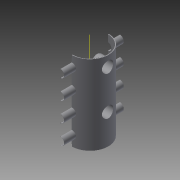
# Autodesk Inventor part: Detection Region Vacuum Collar v2
Saved by Autodesk Inventor 2015 (Build 190159000, 159)
## iProperties
Created: 2014-06-20
Part Number: Detection Region Vacuum Collar v2
Material: Generic
Document SubType Name: Modeling
Designer: Aki
Density: 1 g/cm^3
Appearance: Default
Author: Aki
Autodesk Inventor part; units mm, degrees
ref_plane "XZ Plane" through (0, 0, 0) normal (0, 1, 0) x (-1, 0, 0)
sketch "Sketch1" plane through (0, 0, 0) normal (0, 1, 0) x (-1, 0, 0)
  circle A0 centre (0, 0) radius 101.6
  circle A1 centre (0, 0) radius 97.6
  dimension "d0" = 203.2
  dimension "d3" = 195.2
  constraints: 2 centre point, 2 coincident
  measures "d0" diameter of A0
  measures "d3" diameter of A1
extrude "Extrusion2" add sketch "Sketch1" along normal blind 437.1
ref_plane "Work Plane1" through (0, 0, 101.6) normal (0, 0, 1) x (1, 0, 0)
sketch "Sketch2" plane through (0, 0, 101.6) normal (0, 0, 1) x (1, 0, 0)
  circle A0 centre (0, 57.3) radius 22.25
  circle A1 centre (0, 164.8) radius 22.25
  circle A2 centre (0, 272.3) radius 22.25
  circle A3 centre (0, 379.8) radius 22.25
  line L0 (101.6, 437.1) -> (-101.6, 437.1) projected
  line L1 (-101.6, 0) -> (101.6, 0) projected
  point P0 (0, 0)
  dimension "d7" = 44.5
  dimension "d8" = 44.5
  dimension "d9" = 44.5
  dimension "d10" = 44.5
  dimension "d11" = 57.3
  dimension "d12" = 57.3
  dimension "d13" = 215
  dimension "d14" = 215
  constraints: 4 centre point
  measures "d7" diameter of A0
  measures "d8" diameter of A1
  measures "d9" diameter of A2
  measures "d10" diameter of A3
  measures "d11" distance from line of L0 A3.centre
  measures "d12" distance from line of L1 A0.centre
  measures "d13" distance of A2.centre A0.centre
  measures "d14" distance of A3.centre A1.centre
extrude "Extrusion8" add sketch "Sketch2" against normal up to next
sketch "Sketch13" plane through (0, 0, 101.6) normal (0, 0, 1) x (1, 0, 0)
  circle A0 centre (0, 57.3) radius 22.25
  circle A1 centre (0, 164.8) radius 22.25
  circle A2 centre (0, 272.3) radius 22.25
  circle A3 centre (0, 379.8) radius 22.25
  line L0 (101.6, 437.1) -> (-101.6, 437.1) projected
  line L1 (-101.6, 0) -> (101.6, 0) projected
  point P0 (0, 0)
  dimension "d104" = 44.5
  dimension "d105" = 44.5
  dimension "d106" = 44.5
  dimension "d107" = 44.5
  dimension "d108" = 57.3
  dimension "d109" = 57.3
  dimension "d110" = 215
  dimension "d111" = 215
  constraints: 4 centre point
  measures "d104" diameter of A0
  measures "d105" diameter of A1
  measures "d106" diameter of A2
  measures "d107" diameter of A3
  measures "d108" distance from line of L0 A3.centre
  measures "d109" distance from line of L1 A0.centre
  measures "d110" distance of A2.centre A0.centre
  measures "d111" distance of A3.centre A1.centre
extrude "Extrusion9" add sketch "Sketch13" along normal blind 62.5
ref_plane "Work Plane2" through (0, 0, -101.6) normal (0, 0, 1) x (1, 0, 0)
sketch "Sketch3" plane through (0, 0, -101.6) normal (0, 0, 1) x (1, 0, 0)
  circle A0 centre (0, 57.3) radius 22.25
  circle A1 centre (0, 164.8) radius 22.25
  circle A2 centre (0, 272.3) radius 22.25
  circle A3 centre (0, 379.8) radius 22.25
  line L0 (101.6, 437.1) -> (-101.6, 437.1) projected
  line L1 (-101.6, 0) -> (101.6, 0) projected
  line L2 (0, 357.55) -> (0, 402.05) projected
  point P0 (0, 0)
  dimension "d18" = 44.5
  dimension "d19" = 44.5
  dimension "d20" = 44.5
  dimension "d21" = 44.5
  dimension "d22" = 57.3
  dimension "d23" = 57.3
  dimension "d24" = 215
  dimension "d25" = 215
  dimension "d26" = 0
  constraints: 4 centre point
  measures "d18" diameter of A0
  measures "d19" diameter of A1
  measures "d20" diameter of A2
  measures "d21" diameter of A3
  measures "d22" distance from line of L0 A3.centre
  measures "d23" distance from line of L1 A0.centre
  measures "d24" distance of A0.centre A2.centre
  measures "d25" distance of A3.centre A1.centre
  measures "d26" distance from line of L2 A3.centre
extrude "Extrusion10" add sketch "Sketch3" along normal up to next
sketch "Sketch14" plane through (0, 0, -101.6) normal (0, 0, 1) x (1, 0, 0)
  circle A0 centre (0, 57.3) radius 22.25
  circle A1 centre (0, 164.8) radius 22.25 projected
  circle A2 centre (0, 164.8) radius 22.25
  circle A3 centre (0, 272.3) radius 22.25
  circle A4 centre (0, 379.8) radius 22.25
  line L0 (-101.6, 0) -> (101.6, 0) projected
  line L1 (101.6, 437.1) -> (-101.6, 437.1) projected
  point P0 (0, 0)
  dimension "d116" = 44.5
  dimension "d117" = 44.5
  dimension "d118" = 44.5
  dimension "d119" = 44.5
  dimension "d120" = 57.3
  dimension "d121" = 215
  dimension "d122" = 215
  dimension "d123" = 57.3
  constraints: 4 centre point, 1 coincident
  measures "d116" diameter of A0
  measures "d117" diameter of A2
  measures "d118" diameter of A3
  measures "d119" diameter of A4
  measures "d120" distance from line of L0 A0.centre
  measures "d121" distance of A3.centre A0.centre
  measures "d122" distance of A4.centre A2.centre
  measures "d123" distance from line of L1 A4.centre
extrude "Extrusion11" add sketch "Sketch14" against normal blind 62.5
sketch "Sketch15" plane through (0, 379.8, -164.1) normal (0, 0, -1) x (-1, 0, 0)
  circle A0 centre (0, -322.5106) radius 21.35
  point P0 (0, -379.8)
  dimension "d126" = 42.7
  constraints: 1 centre point
  measures "d126" diameter of A0
hole "Hole8" at (0, 57.2894, -164.1) direction (0, 0, 1) diameter 42.7 end through all
sketch "Sketch16" plane through (0, 164.8, -164.1) normal (0, 0, -1) x (-1, 0, 0)
  circle A0 centre (0, 0) radius 21.35
  point P0 (0, -164.8)
  dimension "d134" = 42.7
  constraints: 1 centre point
  measures "d134" diameter of A0
hole "Hole9" at (0, 164.8, -164.1) direction (0, 0, 1) diameter 42.7 end through all
sketch "Sketch17" plane through (0, 272.3, -164.1) normal (0, 0, -1) x (-1, 0, 0)
  circle A0 centre (0, 0) radius 21.35
  point P0 (0, -272.3)
  dimension "d142" = 42.7
  constraints: 1 centre point
  measures "d142" diameter of A0
hole "Hole10" at (0, 272.3, -164.1) direction (0, 0, 1) diameter 42.7 end through all
sketch "Sketch18" plane through (0, 379.8, -164.1) normal (0, 0, -1) x (-1, 0, 0)
  circle A0 centre (0, 0) radius 21.35
  point P0 (0, -379.8)
  dimension "d150" = 42.7
  constraints: 1 centre point
  measures "d150" diameter of A0
hole "Hole11" at (0, 379.8, -164.1) direction (0, 0, 1) diameter 42.7 end through all
ref_plane "Work Plane3" through (95, 0, 0) normal (1, 0, 0) x (0, 1, 0)
sketch "Sketch19" plane through (95, 0, 0) normal (1, 0, 0) x (0, 1, 0)
  circle A0 centre (164.8, 0) radius 31.75
  circle A1 centre (379.8, 0) radius 31.75
  line L0 (437.1, -101.6) -> (437.1, 101.6) projected
  point P0 (0, 0)
  dimension "d160" = 63.5
  dimension "d161" = 63.5
  dimension "d162" = 215
  dimension "d163" = 57.3
  constraints: 2 centre point
  measures "d160" diameter of A0
  measures "d161" diameter of A1
  measures "d162" distance of A1.centre A0.centre
  measures "d163" distance from line of L0 A1.centre
extrude "Extrusion13" add sketch "Sketch19" along normal up to next
sketch "Sketch20" plane through (95, 0, 0) normal (1, 0, 0) x (0, 1, 0)
  circle A0 centre (164.8, 0) radius 31.75
  circle A1 centre (379.8, 0) radius 31.75
  line L0 (437.1, -101.6) -> (437.1, 101.6) projected
  point P0 (0, 0)
  dimension "d166" = 63.5
  dimension "d167" = 63.5
  dimension "d168" = 215
  dimension "d169" = 57.3
  constraints: 2 centre point
  measures "d166" diameter of A0
  measures "d167" diameter of A1
  measures "d168" distance of A0.centre A1.centre
  measures "d169" distance from line of L0 A1.centre
extrude "Extrusion14" add sketch "Sketch20" against normal blind 55
sketch "Sketch22" plane through (40, 379.8, 0) normal (-1, 0, 0) x (0, 0, 1)
  circle A0 centre (0, 0) radius 30.85
  point P0 (0, -379.8)
  dimension "d180" = 61.7
  constraints: 1 centre point
  measures "d180" diameter of A0
hole "Hole13" at (40, 379.8, 0) direction (1, 0, 0) diameter 61.7 end through all
sketch "Sketch23" plane through (40, 164.8, 0) normal (-1, 0, 0) x (0, 0, 1)
  circle A0 centre (0, 0) radius 30.85
  point P0 (0, -164.8)
  dimension "d188" = 61.7
  constraints: 1 centre point
  measures "d188" diameter of A0
hole "Hole14" at (40, 164.8, 0) direction (1, 0, 0) diameter 61.7 end through all
sketch "Sketch24" plane through (40, 379.8, 0) normal (-1, 0, 0) x (0, 0, 1)
  circle A0 centre (0, 0) radius 30.85 projected
  circle A1 centre (0, 0) radius 29.35
  circle A2 centre (0, 0) radius 30.85
  point P0 (0, -379.8)
  dimension "d196" = 58.7
  dimension "d197" = 61.7
  constraints: 2 centre point, 2 coincident
  measures "d196" diameter of A1
  measures "d197" diameter of A2
extrude "Extrusion15" add sketch "Sketch24" against normal blind 3
sketch "Sketch26" plane through (40, 164.8, 0) normal (-1, 0, 0) x (0, 0, 1)
  circle A0 centre (0, 0) radius 30.85
  circle A1 centre (0, 0) radius 29.35
  point P0 (0, -164.8)
  dimension "d200" = 61.7
  dimension "d201" = 58.7
  constraints: 2 centre point, 1 coincident
  measures "d200" diameter of A0
  measures "d201" diameter of A1
extrude "Extrusion16" add sketch "Sketch26" against normal blind 3
body "Solid2"
